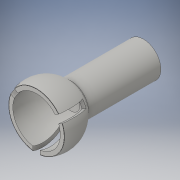
# Autodesk Inventor part: Castor New
Saved by Autodesk Inventor 2016 (Build 200138000, 138)
## iProperties
Created: 2017-09-07
Part Number: Castor New
Material: Generic
Document SubType Name: Modeling
Designer: student
Density: 1 g/cm^3
Appearance: Default
Author: student
Autodesk Inventor part; units mm, degrees
ref_plane "YZ Plane" through (0, 0, 0) normal (1, 0, 0) x (0, 1, 0)
ref_plane "XZ Plane" through (0, 0, 0) normal (0, 1, 0) x (-1, 0, 0)
ref_plane "XY Plane" through (0, 0, 0) normal (0, 0, 1) x (1, 0, 0)
sketch "Sketch1" plane through (0, 0, 0) normal (0, 0, 1) x (1, 0, 0)
  circle A0 centre (0, 0) radius 6.1169
  constraints: 1 centre point, 1 coincident
extrude "Extrusion1" add sketch "Sketch1" along normal blind 25.4
sketch "Sketch2" plane through (0, 0, 0) normal (0, 1, 0) x (-1, 0, 0)
  line L0 (0, 36.9349) -> (0, 25.4)
  line L1 (9.8125, 37.4656) -> (8.5465, 37.4656)
  line L2 (-8.3383, 37.5041) -> (-9.6751, 37.5041)
  line L3 (6.1169, 25.4) -> (-6.1169, 25.4) projected
  line L4 (5.7447, 25.4) -> (-5.7447, 25.4)
  arc A0 (-9.6751, 37.5041) -> (-5.7447, 25.4) centre (0.1507, 34.0045) ccw
  arc A1 (5.7447, 25.4) -> (9.8125, 37.4656) centre (0.1507, 34.0045) ccw
  arc A2 (-8.3383, 37.5041) -> (-3.0546, 25.4) centre (0.1507, 34.0045) ccw
  arc A3 (3.0546, 25.4) -> (8.5465, 37.4656) centre (0.1507, 34.0045) ccw
  point P0 (0, 0)
  dimension "d14" = 9.1821
  constraints: 8 end point, 8 point on circle, 4 centre point, 4 point on line, 2 horizontal, 1 coincident, 1 vertical
  measures "d14" radius of A2
revolve "Revolution1" add sketch "Sketch2" angle 360 about axis through (0, 0, 36.9349) along (0, 0, -1)
sketch "Sketch3" plane through (0, 0, 37.4656) normal (0, 0, 1) x (-1, 0, 0)
  line L0 (0, 0) -> (2.858, 0) construction
  line L1 (0, 0) -> (2.6632, 0) construction
  line L2 (1.27, 10.6058) -> (-1.27, 10.6058)
  line L3 (-1.27, 10.6058) -> (-1.27, 1.4226)
  line L4 (11.2298, -5.0171) -> (1.867, 0.3886)
  line L5 (0.597, -1.8111) -> (9.9598, -7.2168)
  line L6 (9.9598, -7.2168) -> (11.2298, -5.0171)
  circle A0 centre (0, 0) radius 6.1169 projected
  line L7 (-9.6331, -7.0282) -> (-0.597, -1.8111)
  line L8 (-1.867, 0.3886) -> (-10.9031, -4.8285)
  line L9 (-10.9031, -4.8285) -> (-9.6331, -7.0282)
  line L10 (1.27, 1.4226) -> (1.27, 10.6058)
  arc A1 (1.867, 0.3886) -> (1.27, 1.4226) centre (0, 0) ccw
  arc A2 (-1.27, 1.4226) -> (-1.867, 0.3886) centre (0, 0) ccw
  arc A3 (-0.597, -1.8111) -> (0.597, -1.8111) centre (0, 0) ccw
  point P0 (5.2974, -3.0585)
  point P1 (-5.1341, -2.9642)
  dimension "d6" = 2.54
  constraints: 22 end point, 6 point on circle, 3 centre point, 3 parallel, 2 horizontal, 1 coincident, 1 perpendicular, 1 vertical, 2 other
  measures "d6" distance of L2.end L2.start
extrude "Extrusion2" cut sketch "Sketch3" along normal mid plane 18.796 contours L10 A0 L3 L2 | L10 A1 L4 A0 L5 A3 L7 L8 A2 L3 | A0 L7 L9 L8 | L4 L6 L5 A0
sketch "Sketch4" plane through (0, 0, 0) normal (0, 0, -1) x (-1, 0, 0)
  circle A0 centre (0, 0) radius 1.27
  dimension "d13" = 2.54
  constraints: 1 centre point, 1 coincident
  measures "d13" diameter of A0
extrude "Extrusion3" cut sketch "Sketch4" against normal blind 15.24
body "Solid1"
